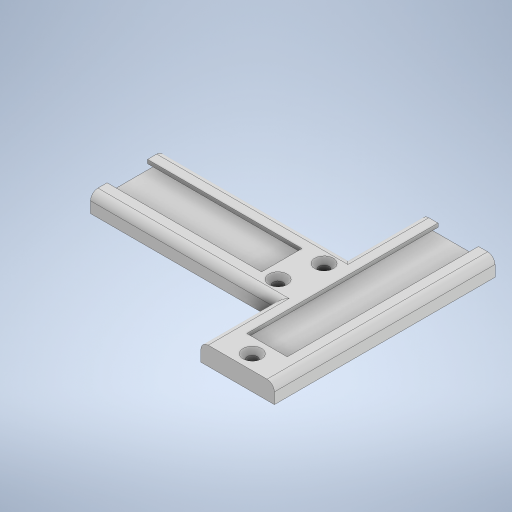
# Autodesk Inventor part: mount1
Saved by Autodesk Inventor 2023 (Build 270158000, 158)
## iProperties
Created: 2025-10-18
Part Number: mount1
Material: Generic
Document SubType Name: Modeling
Designer: Justin Pascual
Density: 1 g/cm^3
Appearance: Default
Mass: 17.3334 g
Surface Area: 113.161 cm^2
Volume: 17.3334 cm^3
Author: Justin Pascual
Autodesk Inventor part; units mm, degrees
ref_plane "YZ Plane" through (0, 0, 0) normal (1, 0, 0) x (0, 1, 0)
ref_plane "XZ Plane" through (0, 0, 0) normal (0, 1, 0) x (-1, 0, 0)
ref_plane "XY Plane" through (0, 0, 0) normal (0, 0, 1) x (1, 0, 0)
sketch "Sketch1" plane through (0, 0, 0) normal (0, 1, 0) x (-1, 0, 0)
  line L0 (0, 0) -> (-88.9, 0)
  line L1 (-88.9, 0) -> (-88.9, -76.2)
  line L2 (-88.9, -76.2) -> (0, -76.2)
  line L3 (0, -76.2) -> (0, 0)
  dimension "d0" = 88.9
  dimension "d1" = 76.2
  constraints: 8 end point, 2 parallel, 1 horizontal, 1 perpendicular
  measures "d0" distance of L2.end L1.end
  measures "d1" distance of L1.end L0.end
extrude "Extrusion1" add sketch "Sketch1" along normal blind 6.35
sketch "Sketch4" plane through (0, 6.35, 0) normal (0, 1, 0) x (1, 0, 0)
  line L0 (0, 76.2) -> (0, 0) projected
  line L1 (0, 0) -> (63.5, 0)
  line L2 (63.5, 0) -> (63.5, 25.4)
  line L3 (63.5, 25.4) -> (0, 25.4)
  line L4 (0, 25.4) -> (0, 0)
  line L5 (0, 76.2) -> (63.5, 76.2)
  line L6 (63.5, 76.2) -> (63.5, 50.8)
  line L7 (63.5, 50.8) -> (0, 50.8)
  line L8 (0, 50.8) -> (0, 76.2)
  point P0 (0, 50.8)
  point P1 (0, 25.4)
  dimension "d4" = 63.5
  dimension "d5" = 63.5
  dimension "d6" = 25.4
  dimension "d7" = 25.4
  constraints: 16 end point, 4 parallel, 2 horizontal, 2 perpendicular
  measures "d4" distance of L3.end L2.end
  measures "d5" distance of L6.end L7.end
  measures "d6" distance between parallel lines of L7 L3
  measures "d7" distance between parallel lines of L1 L3
extrude "Extrusion2" cut sketch "Sketch4" against normal blind 6.35
sketch "Sketch5" plane through (0, 0, -50.8) normal (-1, 0, 0) x (0, 0, 1)
  line L0 (50.8, 6.35) -> (-25.4, 6.35) construction
  line L1 (12.7, 6.35) -> (22.86, 6.35) construction
  line L2 (22.86, 6.35) -> (22.86, 5.08) construction
  line L3 (22.86, 5.08) -> (22.86, 3.175)
  line L4 (22.86, 5.08) -> (19.685, 5.08)
  line L5 (19.685, 5.08) -> (19.685, 6.35) construction
  line L6 (19.685, 5.08) -> (19.685, 3.175) construction
  line L7 (19.685, 3.175) -> (22.86, 3.175)
  line L8 (12.7, 6.35) -> (12.7, 4.445) construction
  line L9 (15.875, 4.572) -> (15.875, 3.175) construction
  line L10 (15.875, 3.175) -> (12.7, 3.175)
  line L11 (12.7, 3.175) -> (12.7, 4.445)
  line L12 (15.875, 6.35) -> (19.685, 6.35)
  line L13 (19.685, 6.35) -> (19.685, 5.08)
  line L14 (19.685, 3.175) -> (15.875, 3.175)
  line L15 (12.7, 4.445) -> (12.7, 6.35)
  line L16 (12.7, 6.35) -> (15.875, 6.35)
  line L17 (-25.4, 6.35) -> (50.8, 6.35) construction
  line L18 (12.7, 6.35) -> (2.54, 6.35) construction
  line L19 (2.54, 6.35) -> (2.54, 5.08) construction
  line L20 (2.54, 5.08) -> (2.54, 3.175)
  line L21 (2.54, 5.08) -> (5.715, 5.08)
  line L22 (5.715, 5.08) -> (5.715, 6.35) construction
  line L23 (5.715, 5.08) -> (5.715, 3.175) construction
  line L24 (5.715, 3.175) -> (2.54, 3.175)
  line L25 (9.525, 4.572) -> (9.525, 3.175) construction
  line L26 (9.525, 3.175) -> (12.7, 3.175)
  line L27 (9.525, 6.35) -> (5.715, 6.35)
  line L28 (5.715, 6.35) -> (5.715, 5.08)
  line L29 (5.715, 3.175) -> (9.525, 3.175)
  line L30 (12.7, 6.35) -> (9.525, 6.35)
  point P0 (50.8, 0)
  dimension "d10" = 10.16
  dimension "d11" = 1.27
  dimension "d12" = 1.905
  dimension "d13" = 3.175
  dimension "d14" = 1.905
  constraints: 60 end point, 11 symmetric about line, 9 point on line, 5 perpendicular, 4 collinear, 3 horizontal, 1 midpoint, 1 vertical
  measures "d10" distance of L1.start L1.end
  measures "d11" distance of L1.end L2.end
  measures "d12" distance of L2.end L3.end
  measures "d13" distance of L2.end L4.end
  measures "d14" distance of L1.start L8.end
extrude "Extrusion3" cut sketch "Sketch5" against normal blind 53.34
sketch "Sketch6" plane through (88.9, 0, -76.2) normal (0, 0, -1) x (-1, 0, 0)
  line L0 (50.8, 6.35) -> (-25.4, 6.35) construction
  line L1 (12.7, 6.35) -> (22.86, 6.35) construction
  line L2 (22.86, 6.35) -> (22.86, 5.08) construction
  line L3 (22.86, 5.08) -> (22.86, 3.175)
  line L4 (22.86, 5.08) -> (19.685, 5.08)
  line L5 (19.685, 5.08) -> (19.685, 6.35) construction
  line L6 (19.685, 5.08) -> (19.685, 3.175) construction
  line L7 (19.685, 3.175) -> (22.86, 3.175)
  line L8 (12.7, 6.35) -> (12.7, 5.08) construction
  line L9 (15.875, 4.572) -> (15.875, 3.175) construction
  line L10 (15.875, 3.175) -> (12.7, 3.175)
  line L11 (12.7, 3.175) -> (12.7, 5.08)
  line L12 (15.875, 6.35) -> (19.685, 6.35)
  line L13 (19.685, 6.35) -> (19.685, 5.08)
  line L14 (19.685, 3.175) -> (15.875, 3.175)
  line L15 (12.7, 5.08) -> (12.7, 6.35)
  line L16 (12.7, 6.35) -> (15.875, 6.35)
  line L17 (2.54, 6.35) -> (2.54, 5.08) construction
  line L18 (2.54, 5.08) -> (2.54, 3.175)
  line L19 (2.54, 5.08) -> (5.715, 5.08)
  line L20 (5.715, 5.08) -> (5.715, 6.35) construction
  line L21 (5.715, 5.08) -> (5.715, 3.175) construction
  line L22 (5.715, 3.175) -> (2.54, 3.175)
  line L23 (5.715, 6.35) -> (5.715, 5.08)
  line L24 (9.525, 4.572) -> (9.525, 3.175) construction
  line L25 (9.525, 6.35) -> (5.715, 6.35)
  line L26 (5.715, 3.175) -> (9.525, 3.175)
  line L27 (9.525, 3.175) -> (12.7, 3.175)
  line L28 (12.7, 6.35) -> (2.54, 6.35) construction
  line L29 (12.7, 6.35) -> (9.525, 6.35)
  line L30 (-25.4, 6.35) -> (50.8, 6.35) construction
  line L31 (0, 6.35) -> (25.4, 6.35) projected
  point P0 (88.9, 0)
  point P1 (50.8, 0)
  dimension "d18" = 10.16
  dimension "d19" = 1.27
  dimension "d20" = 1.905
  dimension "d21" = 3.175
  dimension "d22" = 1.27
  constraints: 62 end point, 11 symmetric about line, 9 point on line, 5 collinear, 5 perpendicular, 3 horizontal, 1 midpoint, 1 vertical
  measures "d18" distance of L1.start L1.end
  measures "d19" distance of L1.end L2.end
  measures "d20" distance of L2.end L3.end
  measures "d21" distance of L2.end L4.end
  measures "d22" distance of L1.start L8.end
extrude "Extrusion4" cut sketch "Sketch6" against normal blind 66.04
sketch "Sketch7" plane through (0, 6.35, 0) normal (0, 1, 0) x (1, 0, 0)
  line L0 (63.5, 50.8) -> (0, 50.8) projected
  line L1 (69.215, 10.16) -> (69.215, 76.2) projected
  line L2 (53.34, 45.085) -> (53.34, 31.115) projected
  line L3 (0, 25.4) -> (63.5, 25.4) projected
  line L4 (63.5, 0) -> (88.9, 0) projected
  line L5 (88.9, 0) -> (88.9, 76.2) projected
  point P0 (0, 0)
  point P1 (61.595, 44.45)
  point P2 (76.2, 5.08)
  point P3 (58.42, 31.75)
  dimension "d25" = 6.35
  dimension "d26" = 7.62
  dimension "d27" = 5.08
  dimension "d28" = 6.35
  dimension "d29" = 5.08
  dimension "d30" = 12.7
  measures "d25" distance from line of L0 point (61.595, 44.45)
  measures "d26" distance from line of L1 point (61.595, 44.45)
  measures "d27" distance from line of L2 point (58.42, 31.75)
  measures "d28" distance from line of L3 point (58.42, 31.75)
  measures "d29" distance from line of L4 point (76.2, 5.08)
  measures "d30" distance from line of L5 point (76.2, 5.08)
hole "Hole1" at (61.595, 6.35, -44.45) at (58.42, 6.35, -31.75) at (76.2, 6.35, -5.08) direction (0, -1, 0) diameter 3.4544 end through all countersink diameter 6.4008 countersink angle 82
fillet "Fillet1" radius 2.54 5 edges at (31.75, 6.35, -50.8) (63.5, 6.35, -63.5) (63.5, 6.35, -12.7) (31.75, 6.35, -25.4) (88.9, 6.35, -38.1)
body "Solid1"
